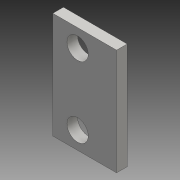
# Autodesk Inventor part: prilozka
Saved by Autodesk Inventor 2016 (Build 200138000, 138)
## iProperties
Created: 2018-11-24
Part Number: prilozka
Material: Generic
Document SubType Name: Modeling
Designer: Radek
Density: 1 g/cm^3
Appearance: Default
Author: Radek
Autodesk Inventor part; units mm, degrees
ref_plane "YZ Plane" through (0, 0, 0) normal (1, 0, 0) x (0, 1, 0)
ref_plane "XZ Plane" through (0, 0, 0) normal (0, 1, 0) x (-1, 0, 0)
ref_plane "XY Plane" through (0, 0, 0) normal (0, 0, 1) x (1, 0, 0)
sketch "Náčrt1" plane through (0, 0, 0) normal (0, 1, 0) x (-1, 0, 0)
  line L0 (0, 0) -> (18, 0)
  line L1 (18, 0) -> (18, -30)
  line L2 (18, -30) -> (0, -30)
  line L3 (0, -30) -> (0, 0)
  circle A0 centre (11, -5) radius 3
  circle A1 centre (11, -25) radius 3
  dimension "d0" = 18
  dimension "d1" = 30
  dimension "d2" = 6
  dimension "d3" = 6
  dimension "d4" = 11
  dimension "d5" = 11
  dimension "d6" = 5
  dimension "d7" = 5
  constraints: 8 end point, 2 centre point, 2 parallel, 1 horizontal, 1 perpendicular
  measures "d0" distance of L1.end L2.end
  measures "d1" distance of L0.end L1.end
  measures "d2" diameter of A0
  measures "d3" diameter of A1
  measures "d4" distance from line of L3 A0.centre
  measures "d5" distance from line of L3 A1.centre
  measures "d6" distance from line of L0 A0.centre
  measures "d7" distance from line of L2 A1.centre
extrude "Vysunutí1" add sketch "Náčrt1" along normal blind 3
equation "\"d5\" = d4"
equation "\"d7\" = d6"
